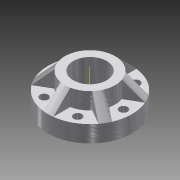
# Autodesk Inventor part: pegg
Saved by Autodesk Inventor 2015 (Build 190159000, 159)
## iProperties
Created: 2016-08-30
Part Number: pegg
Material: Generic
Document SubType Name: Modeling
Designer: ypatel4
Density: 1 g/cm^3
Appearance: Default
Author: ypatel4
Autodesk Inventor part; units mm, degrees
ref_plane "YZ Plane" through (0, 0, 0) normal (1, 0, 0) x (0, 1, 0)
ref_plane "XZ Plane" through (0, 0, 0) normal (0, 1, 0) x (-1, 0, 0)
ref_plane "XY Plane" through (0, 0, 0) normal (0, 0, 1) x (1, 0, 0)
sketch "Sketch1" plane through (0, 0, 0) normal (0, 1, 0) x (-1, 0, 0)
  circle A0 centre (0, 0) radius 12.7
  circle A1 centre (0, 0) radius 31.75
  dimension "d0" = 25.4
  dimension "d1" = 63.5
  constraints: 2 centre point, 2 coincident
  measures "d0" diameter of A0
  measures "d1" diameter of A1
extrude "Extrusion1" add sketch "Sketch1" along normal blind 12.7
sketch "Sketch2" plane through (0, 12.7, 0) normal (0, 1, 0) x (1, 0, 0)
  circle A0 centre (0, 0) radius 19.05
  circle A1 centre (0, 0) radius 31.75 construction
  line L0 (-31.75, 0) -> (-19.05, 0) construction
  circle A2 centre (-25.4, 0) radius 2.5473
  circle A3 centre (0, 0) radius 12.7 projected
  dimension "d5" = 38.1
  constraints: 2 end point, 2 horizontal alignment, 1 centre point, 1 coincident, 1 horizontal, 1 midpoint, 3 other
extrude "Extrusion2" add sketch "Sketch2" along normal blind 12.7 contours A0
sketch "Sketch3" plane through (0, 12.7, 0) normal (0, 1, 0) x (1, 0, 0)
  line L0 (-31.75, 0) -> (-19.05, 0) construction
  circle A0 centre (-25.4, 0) radius 2.5473 projected
  point P0 (0, 0)
hole "Hole1" at (-25.4, 12.7, 0) direction (0, -1, 0) diameter 6.35 end through all
pattern_circular "Circular Pattern1" count 6 over 360 about axis through (0, 0, 0) along (0, 1, 0) of "Hole1"
sketch "Sketch4" plane through (0, 12.7, 0) normal (0, 1, 0) x (1, 0, 0)
  circle A0 centre (0, 0) radius 19.05 projected
  line L0 (3.7235, -18.6826) -> (3.7235, -31.5309)
  arc A1 (-3.7247, -31.5309) -> (3.7235, -31.5309) centre (-0.0006, 0.0104) ccw
  line L1 (-3.7247, -31.5309) -> (-3.7247, -18.6823)
  constraints: 4 end point, 4 point on circle, 1 centre point, 1 vertical
extrude "Extrusion3" add sketch "Sketch4" along normal blind 12.7 contours A0 L0 A1 L1
chamfer "Chamfer1" distance 12.7 angle 45 1 edges at (-0.0006, 25.4, 31.75)
pattern_circular "Circular Pattern2" count 6 over 360 about axis through (0, 0, 0) along (0, 1, 0) of "Extrusion3", "Chamfer1"
